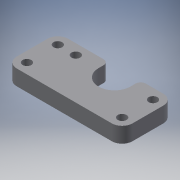
# Autodesk Inventor part: Extruder_clamp
Saved by Autodesk Inventor 2016 (Build 200138000, 138)
## iProperties
Created: 2015-12-28
Part Number: Extruder_clamp
Material: Generic
Document SubType Name: Modeling
Designer: inornate
Density: 1 g/cm^3
Appearance: Default
Author: inornate
Autodesk Inventor part; units mm, degrees
ref_plane "YZ Plane" through (0, 0, 0) normal (1, 0, 0) x (0, 1, 0)
ref_plane "XZ Plane" through (0, 0, 0) normal (0, 1, 0) x (-1, 0, 0)
ref_plane "XY Plane" through (0, 0, 0) normal (0, 0, 1) x (1, 0, 0)
sketch "Sketch1" plane through (0, 0, 0) normal (0, 0, 1) x (1, 0, 0)
  line L0 (8, 8.75) -> (8, 11) construction
  line L1 (8, 11) -> (5.7378, 11) construction
  line L2 (5.7378, 11) -> (5.7378, 8) construction
  line L3 (5.7378, 8) -> (3.2622, 8) construction
  line L4 (3.2622, 8) -> (3.2622, 11) construction
  line L5 (3.2622, 11) -> (-17.2622, 11) construction
  line L6 (-17.2622, 11) -> (-17.2622, 8) construction
  line L7 (-17.2622, 8) -> (-19.7378, 8) construction
  line L8 (-19.7378, 8) -> (-19.7378, 11) construction
  line L9 (-19.7378, 11) -> (-22.75, 11) construction
  line L10 (-25.75, 14) -> (-22.75, 11) construction
  line L11 (-25.75, 14) -> (-25.75, 0) construction
  arc A0 (-25.75, 0) -> (-22, -3.75) centre (-22, 0) ccw construction
  line L12 (-22, -3.75) -> (-20.3954, -3.75) construction
  arc A1 (-16.2094, -6.0156) -> (-20.3954, -3.75) centre (-20.3954, -8.75) ccw construction
  arc A2 (-16.2094, -6.0156) -> (2.2094, -6.0156) centre (-7, 0) ccw construction
  arc A3 (6.3954, -3.75) -> (2.2094, -6.0156) centre (6.3954, -8.75) ccw construction
  line L13 (6.3954, -3.75) -> (8, -3.75) construction
  arc A4 (8, -3.75) -> (11.75, 0) centre (8, 0) ccw construction
  line L14 (11.75, 0) -> (11.75, 7) construction
  line L15 (11.75, 7) -> (9.75, 7) construction
  line L16 (9.75, 7) -> (8, 8.75) construction
  circle A5 centre (-7, 0) radius 8.2 construction
  circle A6 centre (8, 0) radius 1.75 construction
  circle A7 centre (-22, 0) radius 1.75 construction
  circle A8 centre (-22, 0) radius 1.7
  circle A9 centre (8, 0) radius 1.7
  line L17 (-33, 0) -> (-33, -12)
  line L18 (-29, -16) -> (8, -16)
  line L19 (12, -12) -> (12, 0)
  line L20 (15, 5) -> (-29, 5) construction
  circle A10 centre (-29, 0) radius 1.7
  circle A11 centre (-29, -12) radius 1.7
  circle A12 centre (8, -12) radius 1.7
  arc A13 (-29, 4) -> (-33, 0) centre (-29, 0) ccw
  arc A14 (12, 0) -> (8, 4) centre (8, 0) ccw
  arc A15 (8, -16) -> (12, -12) centre (8, -12) ccw
  arc A16 (-33, -12) -> (-29, -16) centre (-29, -12) ccw
  line L21 (-13.2, 0) -> (-13.2, 2)
  line L22 (-0.8, 2) -> (-0.8, 0)
  line L23 (8, 4) -> (1.2, 4)
  line L24 (-15.2, 4) -> (-29, 4)
  arc A17 (-13.2, 0) -> (-0.8, 0) centre (-7, 0) ccw
  arc A18 (1.2, 4) -> (-0.8, 2) centre (1.2, 2) ccw
  arc A19 (-13.2, 2) -> (-15.2, 4) centre (-15.2, 2) ccw
  line L25 (-7, 0) -> (-7, -14.8436)
  circle A20 centre (-29, 0) radius 3 construction
  point P0 (0, 0)
  point P1 (-7, -3)
  dimension "d1" = 3.4
  dimension "d2" = 3.4
  dimension "d7" = 3.4
  dimension "d8" = 3.4
  dimension "d10" = 3.4
  dimension "d11" = 4
  dimension "d13" = 2
  dimension "d16" = 6.2
  dimension "d20" = 37
  dimension "d21" = 12
  dimension "d23" = 4
  dimension "d24" = 6
  constraints: 18 end point, 14 point on circle, 14 tangent, 13 centre point, 7 coincident, 4 equal radius, 4 parallel, 3 perpendicular, 2 horizontal, 1 vertical, 1 vertical alignment
  measures "d1" diameter of A8
  measures "d2" diameter of A9
  measures "d7" diameter of A10
  measures "d8" diameter of A11
  measures "d10" diameter of A12
  measures "d11" radius of A13
  measures "d13" radius of A18
  measures "d16" radius of A17
  measures "d20" distance of A12.centre A11.centre
  measures "d21" distance of A10.centre A11.centre
  measures "d23" distance from line of L25.start L24
  measures "d24" diameter of A20
extrude "Extrusion1" add sketch "Sketch1" along normal blind 6
body "Solid1"
